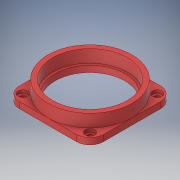
# Autodesk Inventor part: 000.001 - База лидара gjl gjlibgybr
Saved by Autodesk Inventor 2019 (Build 230136000, 136)
## iProperties
Created: 2020-02-21
Part Number: 000.001 - База лидара gjl gjlibgybr
Material: Пластик АБС
Document SubType Name: Modeling
Designer: Петров Иван
Density: 1.06 g/cm^3
Appearance: Гладкий — красный
Author: Петров Иван
Autodesk Inventor part; units mm, degrees
ref_plane "YZ Plane" through (0, 0, 0) normal (1, 0, 0) x (0, 1, 0)
ref_plane "XZ Plane" through (0, 0, 0) normal (0, 1, 0) x (-1, 0, 0)
ref_plane "XY Plane" through (0, 0, 0) normal (0, 0, 1) x (1, 0, 0)
sketch "Эскиз1" plane through (0, 0, 0) normal (0, 1, 0) x (-1, 0, 0)
  circle A0 centre (0, 0) radius 22
  circle A1 centre (0, 0) radius 23.5
  circle A2 centre (0, 0) radius 26.5
  dimension "d0" = 44
  dimension "d1" = 47
  dimension "d2" = 53
  constraints: 3 centre point, 3 coincident
  measures "d0" diameter of A0
  measures "d1" diameter of A1
  measures "d2" diameter of A2
extrude "Выдавливание1" add sketch "Эскиз1" along normal blind 12 contours A2
sketch "Эскиз2" plane through (0, 0, 0) normal (0, -1, 0) x (1, 0, 0)
  circle A0 centre (0, 0) radius 22
  circle A1 centre (0, 0) radius 23.5
  circle A2 centre (0, 0) radius 26.5
  dimension "d5" = 44
  dimension "d6" = 47
  dimension "d7" = 53
  constraints: 3 centre point, 3 coincident
  measures "d5" diameter of A0
  measures "d6" diameter of A1
  measures "d7" diameter of A2
extrude "Выдавливание2" add sketch "Эскиз2" against normal blind 4 contours A1
sketch "Эскиз3" plane through (0, 0, 0) normal (0, -1, 0) x (1, 0, 0)
  circle A0 centre (0, 0) radius 22
  circle A1 centre (0, 0) radius 23.5
  circle A2 centre (0, 0) radius 26.5
  line L0 (-26.5, 26.5) -> (26.5, 26.5)
  line L1 (26.5, 26.5) -> (26.5, -26.5)
  line L2 (26.5, -26.5) -> (-26.5, -26.5)
  line L3 (-26.5, -26.5) -> (-26.5, 26.5)
  line L4 (-26.5, 26.5) -> (26.5, -26.5) construction
  line L5 (26.5, 26.5) -> (-26.5, -26.5) construction
  dimension "d10" = 44
  dimension "d11" = 47
  dimension "d12" = 53
  dimension "d13" = 53
  dimension "d14" = 53
  constraints: 12 end point, 3 centre point, 3 coincident, 2 midpoint, 2 parallel, 1 horizontal, 1 perpendicular
  measures "d10" diameter of A0
  measures "d11" diameter of A1
  measures "d12" diameter of A2
  measures "d13" distance of L1.end L2.end
  measures "d14" distance of L0.end L1.end
extrude "Выдавливание3" add sketch "Эскиз3" against normal blind 4 contours L1 L2 A2 | A2 L0 L1 | A2 L3 L0 | L2 L3 A2
sketch "Эскиз4" plane through (0, 4, 0) normal (0, 1, 0) x (1, 0, 0)
  line L0 (0, 0) -> (21.2132, -21.2132)
  line L1 (0, 0) -> (30, 0) construction
  circle A0 centre (21.2132, -21.2132) radius 1.5
  dimension "d17" = 30
  dimension "d18" = 45
  dimension "d19" = 3
  constraints: 4 end point, 1 centre point, 1 coincident, 1 equal length, 1 horizontal
  measures "d17" distance of L0.start L0.end
  measures "d18" angle of L0 L1
  measures "d19" diameter of A0
extrude "Выдавливание4" cut sketch "Эскиз4" against normal blind 4
pattern_circular "Круговой массив1" count 4 over 360 about axis through (0, -10, 0) along (0, 1, 0) of "Выдавливание4"
sketch "Эскиз5" plane through (0, 4, 0) normal (0, 1, 0) x (1, 0, 0)
  circle A0 centre (21.2132, -21.2132) radius 1.5 projected
  circle A1 centre (21.2132, -21.2132) radius 3
  point P0 (0, 0)
  dimension "d25" = 6
  constraints: 1 centre point, 1 coincident
  measures "d25" diameter of A1
extrude "Выдавливание5" cut sketch "Эскиз5" against normal blind 2
pattern_circular "Круговой массив2" count 4 over 360 about axis through (0, -10, 0) along (0, 1, 0) of "Выдавливание5"
fillet "Сопряжение1" radius 8.5 4 edges at (26.5, 2, -26.5) (26.5, 2, 26.5) (-26.5, 2, -26.5) (-26.5, 2, 26.5)
sketch "Эскиз6" plane through (0, 0, 0) normal (0, -1, 0) x (1, 0, 0)
  arc A0 (-18, 26.5) -> (-26.5, 18) centre (-18, 18) ccw projected
  line L0 (-26.5, -18) -> (-26.5, 18) projected
  arc A1 (-26.5, -18) -> (-18, -26.5) centre (-18, -18) ccw projected
  line L1 (18, -26.5) -> (-18, -26.5) projected
  arc A2 (18, -26.5) -> (26.5, -18) centre (18, -18) ccw projected
  line L2 (26.5, 18) -> (26.5, -18) projected
  arc A3 (26.5, 18) -> (18, 26.5) centre (18, 18) ccw projected
  line L3 (-18, 26.5) -> (18, 26.5) projected
  circle A4 centre (-21.2132, 21.2132) radius 1.5 projected
  circle A5 centre (-21.2132, -21.2132) radius 1.5 projected
  circle A6 centre (21.2132, -21.2132) radius 1.5 projected
  circle A7 centre (21.2132, 21.2132) radius 1.5 projected
  circle A8 centre (0, 0) radius 22 projected
